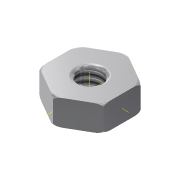
# Autodesk Inventor part: empty
Saved by Autodesk Inventor 2014 (Build 180170000, 170)
## iProperties
Created: 2015-04-13
Part Number: empty
Material: Generic
Document SubType Name: Modeling
Designer: Martin
Density: 1 g/cm^3
Appearance: Default
Author: Martin
Autodesk Inventor part; units mm, degrees
ref_plane "YZ Plane" through (0, 0, 0) normal (1, 0, 0) x (0, 1, 0)
ref_plane "XZ Plane" through (0, 0, 0) normal (0, 1, 0) x (-1, 0, 0)
ref_plane "XY Plane" through (0, 0, 0) normal (0, 0, 1) x (1, 0, 0)
sketch "Sketch1" plane through (0, 0, 0) normal (0, 0, 1) x (1, 0, 0)
  line L0 (0, -3.2332) -> (0, 3.2332) projected
  line L1 (-2.8, 0) -> (2.8, 0) projected
  line L2 (0, 2.3094) -> (-2, 1.1547)
  line L3 (-2, 1.1547) -> (-2, -1.1547)
  line L4 (-2, -1.1547) -> (0, -2.3094)
  line L5 (0, -2.3094) -> (2, -1.1547)
  line L6 (2, -1.1547) -> (2, 1.1547)
  line L7 (2, 1.1547) -> (0, 2.3094)
  circle A0 centre (0, 0) radius 0.74
  point P0 (-2, 0)
  dimension "d2" = 120
  dimension "d3" = 4
  dimension "d6" = 1.48
  constraints: 12 end point, 5 equal length, 3 point on line, 1 centre point, 1 coincident, 1 midpoint, 1 parallel, 1 perpendicular
  measures "d2" angle of L7 L2
  measures "d3" distance between parallel lines of L6 L3
  measures "d6" diameter of A0
extrude "Extrusion2" add sketch "Sketch1" along normal mid plane 1.6
extrude "Extrusion3" cut sketch "Sketch1" along normal through all both and the other way through all contours A0 L1 L0 | L0 L1 A0 | L1 A0 L0 | L0 A0 L1
sketch "Sketch2" plane through (0, 0, 0) normal (1, 0, 0) x (0, 1, 0)
  line L0 (0, -1.1283) -> (0, 1.1697) projected
  line L1 (-2.3094, 0.8) -> (-1.1547, 0.8) projected
  line L2 (-2.3094, -0.8) -> (-2.3094, 0.8) projected
  arc A0 (-2.1094, 0.8) -> (-2.3094, 0.6) centre (-2.1094, 0.6) ccw
  point P0 (0, 0)
  dimension "d14" = 0.2
  constraints: 2 point on circle, 2 point on line, 2 tangent, 1 centre point
  measures "d14" radius of A0
revolve "Revolution1" cut sketch "Sketch2" angle 360 about axis through (0, 0, -10) along (0, 0, 1)
mirror "Mirror1" about plane through (0, 0, 0) normal (0, 0, 1) of "Revolution1"
fillet "Fillet2" radius 0.2 2 edges at (-0.74, 0, -0.8) (-0.74, 0, 0.8)
thread "Thread2" size "M2x0.4" class "6H" standard "ISO Metric profile" full length
body "Solid2"
